Internal Bearing Block_v8 (Autodesk Fusion 360 design; units mm, degrees)
Autodesk Fusion 360 part; units mm, degrees
sketch "Sketch1" plane through (0, 0, 0) normal (1, 0, 0) x (0, 1, 0)
  line L0 (-3.4393, 5.5) -> (-1.8, 5.5)
  line L1 (-12.8393, 3.9) -> (-15.5, 6.5607)
  line L2 (-7.1607, 3.9) -> (-12.8393, 3.9)
  line L3 (-4.5, 6.5607) -> (-7.1607, 3.9)
  line L4 (-4.5, -8.2) -> (-6.7372, -8.2)
  line L5 (-5.5978, 9.8222) -> (-6.8786, 8.5414)
  line L6 (-1.8, 5.5) -> (-1.8, 3.2628)
  line L7 (-19.8494, 4.4312) -> (-18.5414, 3.1214)
  line L8 (-15.5, 8.2) -> (-13.2628, 8.2)
  arc A0 (-5.1686, 10) -> (-5.5978, 9.8222) centre (-5.1686, 9.3929) ccw
  circle A1 centre (-10, 0) radius 2.1
  line L9 (-0.5, 10) -> (-5.1686, 10)
  line L10 (-6.1, 2.8393) -> (-3.4393, 5.5)
  line L11 (-14.8314, 10) -> (-19.5, 10)
  line L12 (0, -9.5) -> (0, -4.8314)
  line L13 (-15.5, -8.2) -> (-15.5, -6.5607)
  line L14 (-15.5, -6.5607) -> (-12.8393, -3.9)
  line L15 (-14.4022, -9.8222) -> (-13.1214, -8.5414)
  line L16 (-19.9987, -4.7917) -> (-20, -9.5)
  line L17 (-18.5414, -3.1214) -> (-19.8222, -4.4022)
  line L18 (-6.8786, -8.5414) -> (-5.7664, -9.6536)
  arc A2 (-19.8222, -4.4022) -> (-19.9987, -4.7917) centre (-19.3929, -4.8314) ccw
  line L19 (-13.9, -2.8393) -> (-16.5607, -5.5)
  line L20 (-16.5607, -5.5) -> (-18.2, -5.5)
  arc A3 (-0.5, -10) -> (0, -9.5) centre (-0.5, -9.5) ccw
  arc A4 (-18.2, -3.2628) -> (-18.5414, -3.1214) centre (-18.4, -3.2628) ccw
  line L21 (-13.2628, -8.2) -> (-15.5, -8.2)
  line L22 (-0.1778, -4.4022) -> (-1.4586, -3.1214)
  arc A5 (-5.7664, -9.6536) -> (-5.1686, -10) centre (-5.1163, -9.2207) ccw
  arc A6 (-20, -9.5) -> (-19.5, -10) centre (-19.5, -9.5) ccw
  line L23 (-1.8, -5.5) -> (-3.4393, -5.5)
  line L24 (-5.1686, -10) -> (-0.5, -10)
  line L25 (-3.4393, -5.5) -> (-6.1, -2.8393)
  line L26 (-12.8393, -3.9) -> (-7.1607, -3.9)
  line L27 (-4.5, -6.5607) -> (-4.5, -8.2)
  arc A7 (0, -4.8314) -> (-0.1778, -4.4022) centre (-0.6071, -4.8314) ccw
  arc A8 (-14.8314, -10) -> (-14.4022, -9.8222) centre (-14.8314, -9.3929) ccw
  line L28 (-18.2, -5.5) -> (-18.2, -3.2628)
  arc A9 (-13.1214, -8.5414) -> (-13.2628, -8.2) centre (-13.2628, -8.4) ccw
  arc A10 (-20, 4.9) -> (-19.8494, 4.4312) centre (-19.3734, 4.8428) ccw
  arc A11 (-13.2628, 8.2) -> (-13.1214, 8.5414) centre (-13.2628, 8.4) ccw
  line L29 (-13.1214, 8.5414) -> (-14.4312, 9.8494)
  arc A12 (-6.8786, 8.5414) -> (-6.7372, 8.2) centre (-6.7372, 8.4) ccw
  arc A13 (-18.5414, 3.1214) -> (-18.2, 3.2628) centre (-18.4, 3.2628) ccw
  arc A14 (-14.4312, 9.8494) -> (-14.8314, 10) centre (-14.8314, 9.3929) ccw
  line L30 (-1.4586, 3.1214) -> (-0.1778, 4.4022)
  line L31 (-15.5, 6.5607) -> (-15.5, 8.2)
  arc A15 (-19.5, 10) -> (-20, 9.5) centre (-19.5, 9.5) ccw
  arc A16 (0, 9.5) -> (-0.5, 10) centre (-0.5, 9.5) ccw
  line L32 (-20, 9.5) -> (-20, 4.9)
  line L33 (-19.5, -10) -> (-14.8314, -10)
  line L34 (-7.1607, -3.9) -> (-4.5, -6.5607)
  line L35 (-1.8, -3.2628) -> (-1.8, -5.5)
  arc A17 (-1.4586, -3.1214) -> (-1.8, -3.2628) centre (-1.6, -3.2628) ccw
  arc A18 (-6.7372, -8.2) -> (-6.8786, -8.5414) centre (-6.7372, -8.4) ccw
  arc A19 (-1.8, 3.2628) -> (-1.4586, 3.1214) centre (-1.6, 3.2628) ccw
  line L36 (0, 4.8314) -> (0, 9.5)
  line L37 (-18.2, 5.5) -> (-16.5607, 5.5)
  line L38 (-13.9, 2.8393) -> (-13.9, -2.8393)
  line L39 (-6.1, -2.8393) -> (-6.1, 2.8393)
  line L40 (-18.2, 3.2628) -> (-18.2, 5.5)
  arc A20 (-0.1778, 4.4022) -> (0, 4.8314) centre (-0.6071, 4.8314) ccw
  line L41 (-4.5, 8.2) -> (-4.5, 6.5607)
  line L42 (-6.7372, 8.2) -> (-4.5, 8.2)
  line L43 (-16.5607, 5.5) -> (-13.9, 2.8393)
  line L44 (-12.7979, 4) -> (-15.4, 6.6021)
  line L45 (-15.4, 6.6021) -> (-15.4, 8.1)
  line L46 (-15.4, 8.1) -> (-13.2628, 8.1)
  arc A21 (-13.2628, 8.1) -> (-13.0509, 8.6124) centre (-13.2628, 8.4) ccw
  line L47 (-13.0509, 8.6124) -> (-14.3627, 9.9223)
  arc A22 (-14.3627, 9.9223) -> (-14.8314, 10.1) centre (-14.8314, 9.3929) ccw
  line L48 (-14.8314, 10.1) -> (-19.5, 10.1)
  arc A23 (-19.5, 10.1) -> (-20.1, 9.5) centre (-19.5, 9.5) ccw
  line L49 (-20.1, 9.5) -> (-20.1, 4.9044)
  arc A24 (-20.1, 4.9044) -> (-19.9226, 4.363) centre (-19.3734, 4.8428) ccw
  line L50 (-19.9226, 4.363) -> (-18.6124, 3.0509)
  arc A25 (-18.6124, 3.0509) -> (-18.1, 3.2628) centre (-18.4, 3.2628) ccw
  line L51 (-18.1, 3.2628) -> (-18.1, 5.4)
  line L52 (-18.1, 5.4) -> (-16.6021, 5.4)
  line L53 (-16.6021, 5.4) -> (-14, 2.7979)
  line L54 (-14, 2.7979) -> (-14, -2.7979)
  line L55 (-14, -2.7979) -> (-16.6021, -5.4)
  line L56 (-16.6021, -5.4) -> (-18.1, -5.4)
  line L57 (-18.1, -5.4) -> (-18.1, -3.2628)
  arc A26 (-18.1, -3.2628) -> (-18.6121, -3.0507) centre (-18.4, -3.2628) ccw
  line L58 (-18.6121, -3.0507) -> (-19.8929, -4.3315)
  arc A27 (-19.8929, -4.3315) -> (-20.0987, -4.7886) centre (-19.3929, -4.8314) ccw
  line L59 (-20.0987, -4.7886) -> (-20.1, -9.4997)
  arc A28 (-20.1, -9.4997) -> (-19.5, -10.1) centre (-19.5, -9.5) ccw
  line L60 (-19.5, -10.1) -> (-14.8314, -10.1)
  arc A29 (-14.8314, -10.1) -> (-14.3315, -9.8929) centre (-14.8314, -9.3929) ccw
  line L61 (-14.3315, -9.8929) -> (-13.0507, -8.6121)
  arc A30 (-13.0507, -8.6121) -> (-13.2628, -8.1) centre (-13.2628, -8.4) ccw
  line L62 (-13.2628, -8.1) -> (-15.4, -8.1)
  line L63 (-15.4, -8.1) -> (-15.4, -6.6021)
  line L64 (-15.4, -6.6021) -> (-12.7979, -4)
  line L65 (-12.7979, -4) -> (-7.2021, -4)
  line L66 (-7.2021, -4) -> (-4.6, -6.6021)
  line L67 (-4.6, -6.6021) -> (-4.6, -8.1)
  line L68 (-4.6, -8.1) -> (-6.7372, -8.1)
  arc A31 (-6.7372, -8.1) -> (-6.9493, -8.6121) centre (-6.7372, -8.4) ccw
  line L69 (-6.9493, -8.6121) -> (-5.8439, -9.7175)
  arc A32 (-5.8439, -9.7175) -> (-5.1718, -10.1) centre (-5.1163, -9.2207) ccw
  line L70 (-5.1718, -10.1) -> (-0.5, -10.1)
  arc A33 (-0.5, -10.1) -> (0.1, -9.5) centre (-0.5, -9.5) ccw
  line L71 (0.1, -9.5) -> (0.1, -4.8314)
  arc A34 (0.1, -4.8314) -> (-0.1071, -4.3315) centre (-0.6071, -4.8314) ccw
  line L72 (-0.1071, -4.3315) -> (-1.3879, -3.0507)
  arc A35 (-1.3879, -3.0507) -> (-1.9, -3.2628) centre (-1.6, -3.2628) ccw
  line L73 (-1.9, -3.2628) -> (-1.9, -5.4)
  line L74 (-1.9, -5.4) -> (-3.3979, -5.4)
  line L75 (-3.3979, -5.4) -> (-6, -2.7979)
  line L76 (-6, -2.7979) -> (-6, 2.7979)
  line L77 (-6, 2.7979) -> (-3.3979, 5.4)
  line L78 (-3.3979, 5.4) -> (-1.9, 5.4)
  line L79 (-1.9, 5.4) -> (-1.9, 3.2628)
  arc A36 (-1.9, 3.2628) -> (-1.3879, 3.0507) centre (-1.6, 3.2628) ccw
  line L80 (-1.3879, 3.0507) -> (-0.1071, 4.3315)
  arc A37 (-0.1071, 4.3315) -> (0.1, 4.8314) centre (-0.6071, 4.8314) ccw
  line L81 (0.1, 4.8314) -> (0.1, 9.5)
  arc A38 (0.1, 9.5) -> (-0.5, 10.1) centre (-0.5, 9.5) ccw
  line L82 (-0.5, 10.1) -> (-5.1686, 10.1)
  arc A39 (-5.1686, 10.1) -> (-5.6685, 9.8929) centre (-5.1686, 9.3929) ccw
  line L83 (-5.6685, 9.8929) -> (-6.9493, 8.6121)
  arc A40 (-6.9493, 8.6121) -> (-6.7372, 8.1) centre (-6.7372, 8.4) ccw
  line L84 (-6.7372, 8.1) -> (-4.6, 8.1)
  line L85 (-4.6, 8.1) -> (-4.6, 6.6021)
  line L86 (-4.6, 6.6021) -> (-7.2021, 4)
  line L87 (-7.2021, 4) -> (-12.7979, 4)
  line L88 (0, -15) -> (0, 15) construction
  line L89 (-0.5, -10) -> (0, -10)
  line L90 (0, -10) -> (26, -10)
  line L91 (26, -10) -> (26, 20)
  line L92 (26, 20) -> (0, 20)
  line L93 (-19.5, 10) -> (0, 20)
  line L94 (13, 20) -> (13, -10) construction
  point P0 (-10, 0)
  dimension "d1" = 0.1
  constraint perpendicular L82 L88
  constraint horizontal L89
  constraint coincident L88 L89.end
  constraint tangent A3 L89
  constraint perpendicular L90 L91
  constraint perpendicular L91 L92
  constraint midpoint L92 L94.start
  constraint midpoint L90 L94.end
extrude "Extrude1" add sketch "Sketch1" along normal blind 26 contours L44 L45 L46 A21 L47 A22 L48 A33 L71 A34 L72 A35 L73 L74 L75 L76 L77 L78 L79 A36 L80 A37 L81 A38 L82 A39 L83 A40 L84 L85 L86 L87 L89 L90 L91 L92 L93
sketch "Sketch2" plane through (0, 0, 20) normal (0, 0, 1) x (-1, 0, 0)
  line L0 (0, -26) -> (0, 0)
  line L1 (0, 0) -> (-26, 0)
  line L2 (-26, 0) -> (-26, -26)
  line L3 (-26, -26) -> (0, -26)
  circle A0 centre (-13, -13) radius 8.05
  circle A1 centre (-13, -13) radius 3
  line L4 (0, -13) -> (-26, -13) construction
  line L5 (-2.15, -13.95) -> (-7.75, -13.95)
  line L6 (-7.75, -13.95) -> (-7.75, -12.05)
  line L7 (-7.75, -12.05) -> (-2.15, -12.05)
  line L8 (-2.15, -12.05) -> (-2.15, -13.95)
  line L9 (-2.15, -13.95) -> (-7.75, -12.05) construction
  line L10 (-7.75, -13.95) -> (-2.15, -12.05) construction
  line L11 (-18.25, -13.95) -> (-23.85, -13.95)
  line L12 (-23.85, -13.95) -> (-23.85, -12.05)
  line L13 (-23.85, -12.05) -> (-18.25, -12.05)
  line L14 (-18.25, -12.05) -> (-18.25, -13.95)
  line L15 (-18.25, -13.95) -> (-23.85, -12.05) construction
  line L16 (-23.85, -13.95) -> (-18.25, -12.05) construction
  point P0 (-4.95, -13)
  point P1 (-21.05, -13)
  dimension "d9" = 16.1
  dimension "d15" = 6
  dimension "d18" = 5.6
  dimension "d19" = 1.9
  dimension "d20" = 5.6
  dimension "d21" = 1.9
  constraint concentric A0 A1
  constraint midpoint L0 L4.start
  constraint midpoint L2 L4.end
  constraint horizontal L5
  constraint perpendicular L5 L6
  constraint parallel L5 L7
  constraint parallel L6 L8
  constraint coincident L9 P0
  constraint coincident L10 P0
  constraint coincident L4 P0
  constraint coincident A0 P0
  constraint horizontal L11
  constraint perpendicular L11 L12
  constraint parallel L11 L13
  constraint parallel L12 L14
  constraint coincident L15 P1
  constraint coincident L16 P1
  constraint coincident A0 P1
  constraint coincident L4 P1
  measures "d9" diameter of A0
  measures "d15" diameter of A1
  measures "d18" distance of L6.end L7.end
  measures "d19" distance of L5.end L6.end
  measures "d20" distance of L12.end L13.end
  measures "d21" distance of L11.end L12.end
extrude "Extrude2" cut sketch "Sketch2" against normal blind 5.1 contours A0 L5 L6 L7 | A0 L5 L6 L7 L11 L13 L14 | A0 L11 L13 L14 | A1
extrude "Extrude3" cut sketch "Sketch2" along normal blind 5.1 from surface at -30 contours A0 L5 L6 L7 | A0 L5 L6 L7 L11 L13 L14 | A0 L11 L13 L14 | A1
extrude "Extrude4" cut sketch "Sketch2" against normal blind 30 contours A1
sketch "Sketch3" plane through (0, 26, 0) normal (0, 1, 0) x (-1, 0, 0)
  line L0 (0, -10) -> (0, 20)
  line L1 (0, 20) -> (-26, 20)
  line L2 (-26, 20) -> (-26, -10)
  line L3 (-26, -10) -> (0, -10)
  line L4 (-27, 0) -> (1, 0) construction
  circle A0 centre (-13, 0) radius 8.05 construction
  circle A1 centre (-21.05, 0) radius 3
  circle A2 centre (-21.05, 0) radius 1.55
  circle A3 centre (-4.95, 0) radius 3
  circle A4 centre (-4.95, 0) radius 1.55
  dimension "d22" = 16.1
  dimension "d23" = 6
  dimension "d24" = 3.1
  dimension "d25" = 6
  dimension "d26" = 3.1
  constraint perpendicular L0 L4
  constraint midpoint L4 A0.centre
  constraint coincident A0 A1.centre
  constraint coincident L4 A1.centre
  constraint concentric A1 A2
  constraint coincident A0 A3.centre
  constraint coincident L4 A3.centre
  constraint concentric A3 A4
  measures "d22" diameter of A0
  measures "d23" diameter of A1
  measures "d24" diameter of A2
  measures "d25" diameter of A3
  measures "d26" diameter of A4
extrude "Extrude5" cut sketch "Sketch3" against normal blind 33 contours A2 | A4
extrude "Extrude6" cut sketch "Sketch3" against normal blind 10 contours A1 | A3
extrude "Extrude7" cut sketch "Sketch2" against normal blind 23 contours A0 L5 L6 L7 | A0 L5 L7 L8 | A0 L11 L13 L14 | A0 L11 L12 L13
